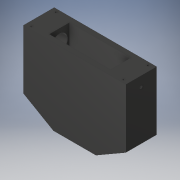
# Autodesk Inventor part: HA01
Saved by Autodesk Inventor 2017 (Build 210142000, 142)
## iProperties
Created: 2018-10-18
Part Number: HA01
Material: ABS Plastic
Document SubType Name: Modeling
Designer: Dell
Density: 1.06 g/cm^3
Appearance: Smooth - Black
Author: Dell
Autodesk Inventor part; units mm, degrees
ref_plane "YZ Plane" through (0, 0, 0) normal (1, 0, 0) x (0, 1, 0)
ref_plane "XZ Plane" through (0, 0, 0) normal (0, 1, 0) x (-1, 0, 0)
ref_plane "XY Plane" through (0, 0, 0) normal (0, 0, 1) x (1, 0, 0)
sketch "Sketch1" plane through (0, 0, 0) normal (0, 0, 1) x (1, 0, 0)
  line L0 (0, -144.3376) -> (-125, -72.1688)
  line L1 (-125, -72.1688) -> (-125, 72.1688)
  line L2 (-125, 72.1688) -> (0, 144.3376) construction
  line L3 (0, 144.3376) -> (125, 72.1688) construction
  line L4 (125, 72.1688) -> (125, -72.1688)
  line L5 (125, -72.1688) -> (0, -144.3376)
  line L6 (125, 72.1688) -> (-125, 72.1688)
  line L7 (125, 72.1688) -> (-125, 72.1688)
  line L8 (-125, 72.1688) -> (-125, 144.3376)
  line L9 (-125, 144.3376) -> (125, 144.3376)
  line L10 (125, 144.3376) -> (125, 72.1688)
  point P0 (0, 0)
  point P1 (0, 0)
  dimension "d0" = 250
  constraints: 22 end point, 2 horizontal, 2 parallel, 2 vertical alignment, 1 coincident, 1 midpoint, 1 perpendicular, 13 other
  measures "d0" distance between parallel lines of L4 L1
extrude "Extrusion1" add sketch "Sketch1" along normal blind 75 contours L0 L1 L6 L4 L5
sketch "Sketch2" plane through (-125, 72.1688, 0) normal (0, 1, 0) x (1, 0, 0)
  line L0 (200, -55) -> (50, -55)
  line L1 (50, -55) -> (50, -20)
  line L2 (50, -20) -> (200, -20)
  line L3 (200, -20) -> (200, -55)
  line L4 (0, 0) -> (0, -75) projected
  line L5 (0, 0) -> (250, 0) projected
  point P0 (125, -20)
  point P1 (50, -37.5)
  point P2 (125, 0)
  point P3 (0, -37.5)
  dimension "d3" = 150
  dimension "d4" = 35
  constraints: 8 end point, 4 midpoint, 2 parallel, 1 horizontal, 1 horizontal alignment, 1 perpendicular, 1 vertical alignment
  measures "d3" distance of L0.start L0.end
  measures "d4" distance of L0.end L1.end
extrude "Extrusion2" cut sketch "Sketch2" against normal through all
sketch "Sketch3" plane through (0, 0, 75) normal (0, 0, 1) x (1, 0, 0)
  line L0 (125, -114.3376) -> (-125, -114.3376)
  line L1 (-125, -114.3376) -> (-125, -144.3376)
  line L2 (-125, -144.3376) -> (125, -144.3376)
  line L3 (125, -144.3376) -> (125, -114.3376)
  point P0 (0, 0)
  point P1 (0, -144.3376)
  point P2 (0, -114.3376)
  point P3 (125, -72.1688)
  dimension "d7" = 30
  constraints: 8 end point, 2 parallel, 2 vertical alignment, 1 horizontal, 1 horizontal alignment, 1 midpoint, 1 perpendicular
  measures "d7" distance of L2.end L0.start
extrude "Extrusion3" cut sketch "Sketch3" against normal through all
sketch "Sketch4" plane through (125, -72.1688, 0) normal (1, 0, 0) x (0, 0, -1)
  circle A0 centre (-37.5, 119.3376) radius 3
  line L0 (0, 144.3376) -> (-75, 144.3376) projected
  point P0 (-37.5, 144.3376)
  dimension "d14" = 6
  dimension "d15" = 25
  constraints: 1 centre point, 1 midpoint, 1 vertical alignment
  measures "d14" diameter of A0
  measures "d15" distance from line of L0 A0.centre
extrude "Extrusion4" cut sketch "Sketch4" against normal through all
sketch "Sketch5" plane through (-125, -72.1688, 0) normal (-1, 0, 0) x (0, 0, 1)
  circle A0 centre (37.5, 119.3376) radius 3 projected
  circle A1 centre (37.5, 112.3376) radius 1.5
  circle A2 centre (53, 112.3376) radius 1.5
  circle A3 centre (45.25, 125.761) radius 1.5
  circle A4 centre (29.75, 125.761) radius 1.5
  circle A5 centre (22, 112.3376) radius 1.5
  circle A6 centre (29.75, 98.9142) radius 1.5
  circle A7 centre (45.25, 98.9142) radius 1.5
  circle A8 centre (37.5, 119.3376) radius 6
  point P0 (0, 72.1688)
  dimension "d16" = 3
  dimension "d17" = 3
  dimension "d18" = 7
  dimension "d19" = 15.5
  dimension "d22" = 360
  dimension "d26" = 12
  constraints: 8 centre point, 1 coincident, 1 horizontal alignment, 1 vertical alignment, 13 other
  measures "d16" diameter of A1
  measures "d17" diameter of A2
  measures "d18" distance of A0.centre A1.centre
  measures "d19" distance of A1.centre A2.centre
  measures "d26" diameter of A8
extrude "Extrusion5" cut sketch "Sketch5" against normal blind 75 contours A0 | A8 A1 | A1 A8 | A2 | A3 | A4 | A5 | A6 | A7 picked at (37.446, 113.508) picked at (36.0874, 114.6648)
sketch "Sketch6" plane through (-75, 72.1688, 55) normal (1, 0, 0) x (0, 0, -1)
  circle A0 centre (17.5, -32) radius 20
  circle A1 centre (33, -32) radius 1.5 projected
  circle A2 centre (17.5, -25) radius 6 projected
  point P0 (55, -72.1688)
  dimension "d27" = 40
  constraints: 1 centre point, 1 horizontal alignment, 1 vertical alignment
  measures "d27" diameter of A0
extrude "Extrusion6" cut sketch "Sketch6" along normal blind 150 and the other way blind 45 contours A0 | A1 | A2
sketch "Sketch7" plane through (-125, 72.1688, 0) normal (0, 1, 0) x (1, 0, 0)
  line L0 (50, -12.5) -> (200, -12.5)
  line L1 (200, -12.5) -> (200, -62.5)
  line L2 (200, -62.5) -> (50, -62.5)
  line L3 (50, -62.5) -> (50, -12.5)
  line L4 (50, -55) -> (50, -20) projected
  line L5 (200, -20) -> (200, -55) projected
  point P0 (125, 0)
  point P1 (50, -37.5)
  dimension "d32" = 50
  constraints: 8 end point, 2 midpoint, 2 parallel, 2 vertical alignment, 1 horizontal, 1 perpendicular
  measures "d32" distance of L2.end L0.start
extrude "Extrusion7" cut sketch "Sketch7" against normal blind 50
sketch "Sketch8" plane through (-125, 72.1688, 0) normal (0, 1, 0) x (1, 0, 0)
  line L0 (12.5, -7.5) -> (237.5, -7.5) construction
  line L1 (237.5, -7.5) -> (237.5, -67.5) construction
  line L2 (237.5, -67.5) -> (12.5, -67.5) construction
  line L3 (12.5, -67.5) -> (12.5, -7.5) construction
  line L4 (50, -62.5) -> (50, -12.5) construction
  line L5 (50, -12.5) -> (200, -12.5) construction
  circle A0 centre (12.5, -7.5) radius 2.5
  circle A1 centre (12.5, -67.5) radius 2.5
  circle A2 centre (237.5, -67.5) radius 2.5
  circle A3 centre (237.5, -7.5) radius 2.5
  point P0 (125, 0)
  point P1 (125, -12.5)
  point P2 (125, -12.5)
  point P3 (125, -7.5)
  point P4 (50, -37.5)
  point P5 (12.5, -37.5)
  dimension "d35" = 225
  dimension "d36" = 60
  dimension "d37" = 5
  dimension "d38" = 5
  dimension "d39" = 5
  dimension "d40" = 5
  constraints: 8 end point, 5 midpoint, 4 centre point, 4 coincident, 2 parallel, 1 horizontal, 1 horizontal alignment, 1 perpendicular, 1 vertical alignment
  measures "d35" distance of L0.start L0.end
  measures "d36" distance of L2.end L0.start
  measures "d37" diameter of A0
  measures "d38" diameter of A1
  measures "d39" diameter of A2
  measures "d40" diameter of A3
extrude "Extrusion8" cut sketch "Sketch8" against normal blind 50
sketch "Sketch9" plane through (-125, -72.1688, 0) normal (-1, 0, 0) x (0, 0, 1)
  circle A0 centre (22, 112.3376) radius 1.5 construction
  circle A1 centre (37.5, 119.3376) radius 3 construction
  line L0 (22, 112.3376) -> (37.5, 112.3376) construction
  circle A2 centre (37.5, 119.3376) radius 6 construction
  line L1 (37.5, 112.3376) -> (37.5, 119.3376) construction
  circle A3 centre (22, 112.3376) radius 4
  circle A4 centre (29.75, 98.9142) radius 4
  circle A5 centre (45.25, 98.9142) radius 4
  circle A6 centre (53, 112.3376) radius 4
  circle A7 centre (45.25, 125.761) radius 4
  circle A8 centre (29.75, 125.761) radius 4
  point P0 (0, 72.1688)
  dimension "d43" = 8
  dimension "d46" = 360
  constraints: 6 centre point, 4 end point, 1 coincident, 1 horizontal, 1 perpendicular, 13 other
  measures "d43" diameter of A3
extrude "Extrusion9" cut sketch "Sketch9" against normal blind 2
body "Solid1"
